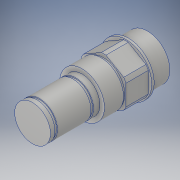
# Autodesk Inventor part: Powered Pivot
Saved by Autodesk Inventor 2019.4 (Build 234330000, 330)
## iProperties
Created: 2020-01-12
Part Number: Powered Pivot
Material: Aluminum 6061
Document SubType Name: Modeling
Designer: admin
Density: 2.7 g/cm^3
Appearance: Aluminum - Flat
Author: admin
Autodesk Inventor part; units mm, degrees
ref_plane "YZ Plane" through (0, 0, 0) normal (1, 0, 0) x (0, 1, 0)
ref_plane "XZ Plane" through (0, 0, 0) normal (0, 1, 0) x (-1, 0, 0)
ref_plane "XY Plane" through (0, 0, 0) normal (0, 0, 1) x (1, 0, 0)
sketch "Sketch1" plane through (0, 0, 0) normal (1, 0, 0) x (0, 1, 0)
  line L0 (0, 0) -> (8, 0)
  line L1 (8, 0) -> (8, -2)
  line L2 (8, -2) -> (7.6, -2)
  line L3 (7.6, -2) -> (7.6, -3.1)
  line L4 (7.6, -3.1) -> (8, -3.1)
  line L5 (9.5, -31.7) -> (11, -31.7)
  line L6 (11, -41.7) -> (11.5, -41.7)
  line L7 (11.5, -41.7) -> (11.5, -42.8)
  line L8 (11.5, -42.8) -> (10, -42.8)
  line L9 (10, -42.8) -> (10, -51.3)
  line L10 (10, -51.3) -> (0, -51.3)
  line L11 (0, -51.3) -> (0, 0)
  line L12 (11, -41.7) -> (11, -31.7)
  line L13 (9.5, -31.7) -> (9.5, -30.6)
  line L14 (9.5, -30.6) -> (10, -30.6)
  line L15 (10, -30.6) -> (10, -22.1)
  line L16 (10, -22.1) -> (8, -22.1)
  line L17 (8, -22.1) -> (8, -19.2)
  line L18 (8, -19.2) -> (7.6, -19.2)
  line L19 (7.6, -19.2) -> (7.6, -18.1)
  line L20 (7.6, -18.1) -> (8, -18.1)
  line L21 (8, -18.1) -> (8, -3.1)
  dimension "d18" = 0.4
  dimension "d19" = 1.1
  dimension "d21" = 2
  dimension "d22" = 8
  dimension "d24" = 10
  dimension "d25" = 1.1
  dimension "d26" = 8.5
  dimension "d27" = 11
  dimension "d28" = 1.5
  dimension "d30" = 0.5
  dimension "d31" = 1.1
  dimension "d32" = 1.1
  dimension "d33" = 0.4
  dimension "d34" = 15
  dimension "d35" = 8.5
  dimension "d36" = 10
  dimension "d37" = 4
  constraints: 44 end point, 16 perpendicular, 2 horizontal, 2 point on line, 1 collinear, 1 vertical
  measures "d18" distance of L3.end L4.end
  measures "d19" distance of L2.end L3.end
  measures "d21" distance of L0.end L1.end
  measures "d22" distance between parallel lines of L11 L1
  measures "d24" distance between parallel lines of L11 L9
  measures "d25" distance of L6.end L7.end
  measures "d26" distance of L8.end L9.end
  measures "d27" distance between parallel lines of L11 L12
  measures "d28" distance of L7.end L8.end
  measures "d30" distance of L13.end L14.end
  measures "d31" distance of L5.start L13.end
  measures "d32" distance of L18.end L19.end
  measures "d33" distance of L17.end L18.end
  measures "d34" distance of L20.end L4.end
  measures "d35" distance of L14.end L15.end
  measures "d36" distance of L6.start L5.end
  measures "d37" distance between parallel lines of L16 L20
revolve "Revolution1" add sketch "Sketch1" angle 360 about axis through (0, 0, -51.3) along (0, 0, 1)
sketch "Sketch2" plane through (0, 0, -31.7) normal (0, 0, 1) x (1, 0, 0)
  circle A0 centre (0, 0) radius 11 projected
  line L0 (0, 11.547) -> (1.0314, 10.9515)
  line L1 (10, 5.7735) -> (10, 4.5826)
  line L2 (10, -5.7735) -> (8.9686, -6.369)
  line L3 (0, -11.547) -> (-1.0314, -10.9515)
  line L4 (-10, -5.7735) -> (-10, -4.5826)
  line L5 (-10, 5.7735) -> (-8.9686, 6.369)
  circle A1 centre (0, 0) radius 10
  line L6 (-8.9686, 6.369) -> (-1.0314, 10.9515)
  line L7 (-10, 4.5826) -> (-10, 5.7735)
  line L8 (-1.0314, 10.9515) -> (0, 11.547)
  line L9 (1.0314, 10.9515) -> (8.9686, 6.369)
  line L10 (8.9686, 6.369) -> (10, 5.7735)
  line L11 (10, 4.5826) -> (10, -4.5826)
  line L12 (10, -4.5826) -> (10, -5.7735)
  line L13 (8.9686, -6.369) -> (1.0314, -10.9515)
  line L14 (-1.0314, -10.9515) -> (-8.9686, -6.369)
  line L15 (1.0314, -10.9515) -> (0, -11.547)
  line L16 (-8.9686, -6.369) -> (-10, -5.7735)
  line L17 (-10, -4.5826) -> (-10, 4.5826)
  point P0 (0, 0)
  dimension "d38" = 20
  constraints: 36 end point, 3 tangent, 2 coincident, 1 centre point, 26 other
  measures "d38" diameter of A1
extrude "Extrusion1" cut sketch "Sketch2" against normal up to surface (10 mm away) contours A0 L11 | L9 A0 | A0 L13 | L6 A0 | L14 A0 | L17 A0
body "Solid1"
